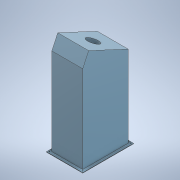
# Autodesk Inventor part: Base
Saved by Autodesk Inventor 2022 (Build 260153000, 153)
## iProperties
Created: 2021-04-24
Part Number: Base
Material: Generic
Document SubType Name: Modeling
Designer: Mick Veldhuis
Density: 1 g/cm^3
Appearance: Default
Author: Mick Veldhuis
Autodesk Inventor part; units mm, degrees
ref_plane "YZ Plane" through (0, 0, 0) normal (1, 0, 0) x (0, 1, 0)
ref_plane "XZ Plane" through (0, 0, 0) normal (0, 1, 0) x (-1, 0, 0)
ref_plane "XY Plane" through (0, 0, 0) normal (0, 0, 1) x (1, 0, 0)
sketch "Sketch1" plane through (0, 0, 0) normal (0, 1, 0) x (-1, 0, 0)
  line L0 (200, 280) -> (-200, 280)
  line L1 (-200, 280) -> (-200, -280)
  line L2 (-200, -280) -> (200, -280)
  line L3 (200, -280) -> (200, 280)
  line L4 (200, 280) -> (-200, -280) construction
  line L5 (-200, 280) -> (200, -280) construction
  point P0 (0, 0)
  constraints: 12 end point, 2 midpoint, 2 parallel, 1 horizontal, 1 perpendicular
extrude "Base" add sketch "Sketch1" along normal blind 5
sketch "Sketch3" plane through (0, 5, 0) normal (0, 1, 0) x (1, 0, 0)
  line L0 (-170, -250) -> (170, -250)
  line L1 (170, -250) -> (170, 250)
  line L2 (170, 250) -> (-170, 250)
  line L3 (-170, 250) -> (-170, -250)
  line L4 (-170, -250) -> (170, 250) construction
  line L5 (170, -250) -> (-170, 250) construction
  point P0 (0, 0)
  constraints: 12 end point, 2 midpoint, 2 parallel, 1 horizontal, 1 perpendicular
extrude "Stand" add sketch "Sketch3" along normal blind 900
move faces "Move2" translate (0, 200.25, 0) faces at (56.6667, 905, 83.3333)
chamfer "FrontChamfer" distance 140 angle 25 1 edges at (0, 1105.25, 250) measured on face at (-56.6667, 371.75, 250)
chamfer "BeamHoleFace" distance 202.7 angle 65 1 edges at (0, 1105.25, -250) measured on face at (56.6667, 371.75, -250)
sketch "Sketch5" plane through (-170, 1105.25, 184.6916) normal (0, 0.9063078, -0.4226183) x (1, 0, 0)
  circle A0 centre (170, 239.8145) radius 65
  point P0 (170, 634.4862)
  point P1 (170, 240)
  point P2 (170, 240)
  point P3 (203, 347)
  point P4 (170, 240)
  constraints: 4 coincident, 1 centre point
extrude "BeamHole" cut sketch "Sketch5" against normal blind 200
sketch "Sketch6" plane through (0, 5, 0) normal (0, 1, 0) x (1, 0, 0)
  circle A0 centre (-184, -264) radius 5
  circle A1 centre (184, -264) radius 5
  line L0 (200, -280) -> (200, 280) construction
  line L1 (200, 0) -> (-200, 0) construction
  line L2 (-200, 280) -> (-200, -280) construction
  circle A2 centre (-184, 264) radius 5
  circle A3 centre (184, 264) radius 5
  point P0 (0, 0)
  constraints: 4 centre point, 2 end point, 2 midpoint, 2 symmetric about line, 2 other
extrude "BaseBoltHoles" cut sketch "Sketch6" against normal up to next
